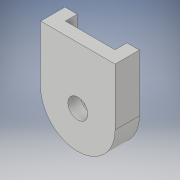
# Autodesk Inventor part: new jewel fail
Saved by Autodesk Inventor 2017 (Build 210142000, 142)
## iProperties
Created: 2018-01-26
Part Number: new jewel fail
Material: Generic
Document SubType Name: Modeling
Designer: Delta
Density: 1 g/cm^3
Appearance: Default
Author: Delta
Autodesk Inventor part; units mm, degrees
ref_plane "YZ Plane" through (0, 0, 0) normal (1, 0, 0) x (0, 1, 0)
ref_plane "XZ Plane" through (0, 0, 0) normal (0, 1, 0) x (-1, 0, 0)
ref_plane "XY Plane" through (0, 0, 0) normal (0, 0, 1) x (1, 0, 0)
sketch "Sketch1" plane through (0, 0, 0) normal (0, 0, 1) x (1, 0, 0)
  line L0 (0, 0) -> (12.7, 0)
  line L1 (12.7, 0) -> (12.7, -11.43)
  line L2 (6.35, -17.78) -> (6.35, -17.78)
  line L3 (0, -11.43) -> (0, 0)
  arc A0 (6.35, -17.78) -> (12.7, -11.43) centre (6.35, -11.43) ccw
  arc A1 (0, -11.43) -> (6.35, -17.78) centre (6.35, -11.43) ccw
  point P0 (12.7, -17.78)
  point P1 (0, -17.78)
  dimension "d0" = 12.7
  dimension "d1" = 17.78
  dimension "d2" = 6.35
  constraints: 8 end point, 4 point on circle, 4 point on line, 4 tangent, 2 centre point, 2 parallel, 1 concentric, 1 horizontal, 1 perpendicular
  measures "d0" distance of point (12.7, -17.78) point (0, -17.78)
  measures "d1" distance of L0.end point (12.7, -17.78)
  measures "d2" radius of A0
extrude "Extrusion1" add sketch "Sketch1" along normal blind 3.175
sketch "Sketch2" plane through (0, 0, 3.175) normal (0, 0, 1) x (1, 0, 0)
  line L0 (12.7, 0) -> (0, 0) projected
  line L1 (0, 0) -> (0, -11.43) projected
  arc A0 (0, -11.43) -> (12.7, -11.43) centre (6.35, -11.43) ccw projected
  line L2 (12.7, -11.43) -> (12.7, 0) projected
  line L3 (-3.175, 3.175) -> (15.875, 3.175)
  line L4 (15.875, 3.175) -> (15.875, -11.43)
  arc A1 (-3.175, -11.43) -> (15.875, -11.43) centre (6.35, -11.43) ccw
  line L5 (-3.175, -11.43) -> (-3.175, 3.175)
  dimension "d5" = 3.175
  constraints: 6 end point, 2 point on circle, 1 centre point, 3 other
  measures "d5" distance between parallel lines of L0 L3
extrude "Extrusion2" add sketch "Sketch2" against normal blind 6.223
sketch "Sketch3" plane through (0, 0, -3.048) normal (0, 0, -1) x (-1, 0, 0)
  line L0 (-15.875, 3.175) -> (-15.875, -11.43) projected
  line L1 (-15.875, 3.175) -> (3.351, 3.175)
  line L2 (3.351, 3.175) -> (3.351, 0)
  line L3 (3.351, 0) -> (-15.875, 0)
  line L4 (-15.875, 0) -> (-15.875, 3.175)
  line L5 (-12.7, 0) -> (0, 0) projected
  line L6 (3.175, 3.175) -> (-15.875, 3.175) projected
  line L7 (-12.7, 0) -> (0, 0)
  line L8 (0, 0) -> (0, 3.175)
  line L9 (0, 3.175) -> (-12.7, 3.175)
  line L10 (-12.7, 3.175) -> (-12.7, 0)
  constraints: 16 end point, 4 parallel, 2 horizontal, 2 perpendicular, 1 point on line
extrude "Extrusion3" cut sketch "Sketch3" against normal blind 3.048 contours L1 L8 L3 L10
sketch "Sketch4" plane through (0, 0, 0) normal (0, 0, -1) x (-1, 0, 0)
  arc A0 (-12.7, -11.43) -> (0, -11.43) centre (-6.35, -11.43) ccw projected
  circle A1 centre (-6.35, -11.43) radius 2.54
  point P0 (0, 0)
  dimension "d10" = 5.08
  constraints: 1 centre point, 1 coincident
  measures "d10" diameter of A1
extrude "Extrusion4" cut sketch "Sketch4" against normal blind 25.4
body "Solid1"
